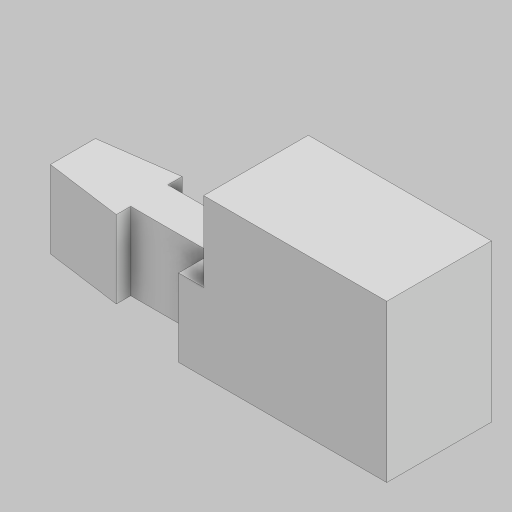
# Autodesk Inventor part: Tenon_Macho_Parametrizado
Saved by Autodesk Inventor 2023 (Build 270158000, 158)
## iProperties
Created: 2026-02-15
Part Number: Tenon_Macho_Parametrizado
Material: Genérico
Document SubType Name: Modeling
Designer: MARTIN MAESTRE
Density: 1 g/cm^3
Appearance: Valor por defecto
Author: MARTIN MAESTRE
Autodesk Inventor part; units mm, degrees
ref_plane "YZ Plane" through (0, 0, 0) normal (1, 0, 0) x (0, 1, 0)
ref_plane "XZ Plane" through (0, 0, 0) normal (0, 1, 0) x (-1, 0, 0)
ref_plane "XY Plane" through (0, 0, 0) normal (0, 0, 1) x (1, 0, 0)
sketch "Boceto1" plane through (0, 0, 0) normal (0, 0, 1) x (1, 0, 0)
  line L0 (0, 0) -> (140, 0)
  line L1 (140, 0) -> (140, 60)
  line L2 (140, 60) -> (0, 60)
  line L3 (0, 60) -> (0, 0)
  dimension "d0" = 140
  dimension "d1" = 60
  constraints: 8 end point, 3 perpendicular, 1 horizontal
  measures "d0" distance of L0.start L0.end
  measures "d1" distance of L0.end L1.end
extrude "Extrusión1" add sketch "Boceto1" along normal blind 40
sketch "Boceto2" plane through (0, 60, 0) normal (0, 1, 0) x (1, 0, 0)
  line L0 (140, -40) -> (0, -40) projected
  line L1 (0, 0) -> (0, -40)
  line L2 (140, 0) -> (0, 0) projected
  line L3 (0, 0) -> (70, 0)
  line L4 (0, 0) -> (70, 0) construction
  line L5 (70, 0) -> (70, -40)
  line L6 (0, -40) -> (70, -40)
  point P0 (70, 0)
  dimension "d4" = 70
  dimension "d5" = 0
  constraints: 10 end point, 3 collinear, 1 horizontal, 1 midpoint, 1 vertical
  measures "d4" distance of L1.start L3.end
  measures "d5" distance between parallel lines of L3 L4
extrude "Extrusión2" cut sketch "Boceto2" against normal blind 30.4
sketch "Boceto3" plane through (0, 0, 0) normal (0, -1, 0) x (1, 0, 0)
  line L0 (0, 0) -> (140, 0) projected
  line L1 (0, 0) -> (0, 11.4)
  line L2 (0, 0) -> (0, 40) projected
  line L3 (0, 11.4) -> (0, 28.6) construction
  line L4 (0, 28.6) -> (0, 40)
  line L5 (0, 0) -> (29.2, 0)
  line L6 (29.2, 0) -> (29.2, 7.4) construction
  line L7 (0, 11.4) -> (29.2, 7.4)
  line L8 (29.2, 0) -> (29.2, 7.4)
  line L9 (29.2, 7.4) -> (29.2, 12.9)
  line L10 (29.2, 12.9) -> (60.4, 12.9)
  line L11 (29.2, 0) -> (60.4, 0)
  line L12 (60.4, 0) -> (60.4, 12.9)
  line L13 (0, 40) -> (140, 40) projected
  line L14 (0, 40) -> (60.4, 40)
  line L15 (60.4, 40) -> (60.4, 27.1)
  line L16 (60.4, 27.1) -> (29.2, 27.1)
  line L17 (60.4, 27.1) -> (91.6, 27.1) construction
  line L18 (29.2, 27.1) -> (29.2, 32.6)
  line L19 (29.2, 32.6) -> (0, 28.6)
  dimension "d8" = 11.4
  dimension "d9" = 17.2
  dimension "d10" = 29.2
  dimension "d11" = 7.4
  dimension "d12" = 5.5
  dimension "d13" = 31.2
  dimension "d14" = 12.9
  dimension "d15" = 60.4
  dimension "d16" = 31.2
  dimension "d17" = 180
  dimension "d18" = 5.5
  constraints: 34 end point, 5 point on line, 4 perpendicular, 3 vertical, 2 collinear, 2 horizontal
  measures "d8" distance of L0.start L1.end
  measures "d9" distance of L1.end L3.end
  measures "d10" distance of L0.start L5.end
  measures "d11" distance of L5.end L6.end
  measures "d12" distance of L6.end L9.end
  measures "d13" distance of L9.end L10.end
  measures "d14" distance of L14.end L15.end
  measures "d15" distance between parallel lines of L2 L15
  measures "d16" distance of L15.end L16.end
  measures "d17" angle of L16 L17
  measures "d18" distance of L16.end L18.end
extrude "Extrusión3" cut sketch "Boceto3" against normal blind 30
equation "\"d4\" = Largo_mitad"
equation "\"d12\" = Prof_corte"
equation "\"d18\" = Prof_corte"
equation "\"Largo_mitad\" = 70"
equation "\"Prof_corte\" = 5.5"
equation "\"Separacion_1\" = 11"
equation "\"Separacion_2\" = 7"
equation "\"Separacion_3\" = 12.5"
equation "\"Angulo_0\" = 0"
equation "\"Angulo_180\" = 180deg"
